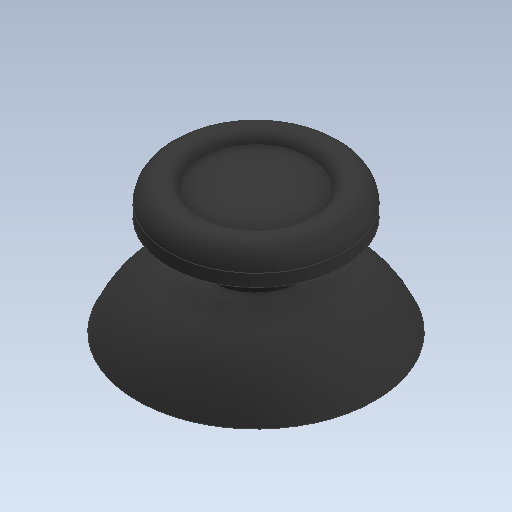
# Autodesk Inventor part: Joystick Cap
Saved by Autodesk Inventor 2020 (Build 240168000, 168)
## iProperties
Created: 2021-03-29
Part Number: Joystick Cap
Material: Generic
Document SubType Name: Modeling
Designer: Luke
Density: 1 g/cm^3
Appearance: Default
Author: Luke
Autodesk Inventor part; units mm, degrees
ref_plane "YZ Plane" through (0, 0, 0) normal (1, 0, 0) x (0, 1, 0)
ref_plane "XZ Plane" through (0, 0, 0) normal (0, 1, 0) x (-1, 0, 0)
ref_plane "XY Plane" through (0, 0, 0) normal (0, 0, 1) x (1, 0, 0)
sketch "Sketch1" plane through (0, 0, 0) normal (0, 1, 0) x (-1, 0, 0)
  line L0 (1.3229, -1.5) -> (-1.3229, -1.5)
  line L1 (-1.3229, 1.5) -> (1.3229, 1.5)
  arc A0 (1.3229, -1.5) -> (1.3229, 1.5) centre (0, 0) ccw
  arc A1 (-1.3229, 1.5) -> (-1.3229, -1.5) centre (0, 0) ccw
  circle A2 centre (0, 0) radius 4.67
  dimension "d1" = 9.34
  constraints: 4 end point, 4 point on circle, 3 centre point, 1 coincident, 1 horizontal, 1 parallel
  measures "d1" diameter of A2
extrude "Extrusion1" add sketch "Sketch1" along normal blind 3.6
sketch "Sketch2" plane through (0, 0, 0) normal (0, 0, 1) x (1, 0, 0)
  line L0 (4.67, 3.6) -> (-4.67, 3.6) projected
  line L1 (0, 3.6) -> (9.08, 3.6)
  line L2 (0, 3.6) -> (9.08, 3.6) construction
  line L3 (0, 3.6) -> (0, 6.9)
  line L4 (9.08, 4.9) -> (9.08, 3.461)
  arc A0 (9.08, 4.9) -> (7.08, 6.9) centre (7.08, 4.9) ccw
  line L5 (0, 6.9) -> (0, 6.17)
  arc A1 (7.08, 6.9) -> (5.535, 6.17) centre (7.08, 4.9) ccw
  arc A2 (5.535, 6.17) -> (0, 6.535) centre (0.5987, -26.5352) ccw
  point P0 (0, 6.535)
  dimension "d5" = 9.08
  dimension "d8" = 3.3
  dimension "d9" = 2
  dimension "d10" = 0.73
  constraints: 10 end point, 7 point on circle, 3 centre point, 2 horizontal, 2 midpoint, 1 concentric, 1 perpendicular, 1 point on line, 1 tangent, 1 vertical
  measures "d5" distance of L1.start L1.end
  measures "d8" distance of L1.start L3.end
  measures "d9" radius of A0
  measures "d10" distance of L3.end L5.end
revolve "Revolution1" add sketch "Sketch2" angle 360 about axis through (0, 3.6, 0) along (0, 1, 0)
sketch "Sketch3" plane through (0, 0, 0) normal (0, 0, 1) x (1, 0, 0)
  arc A0 (12.4, -6.81) -> (4.67, 0) centre (1.8593, -10.9825) ccw
  arc A1 (11.1849, -6.81) -> (4.3923, -1.085) centre (1.8593, -10.9825) ccw
  line L0 (12.4, -6.81) -> (11.1849, -6.81)
  line L1 (2, 0) -> (2, -1.085)
  line L2 (2, -1.085) -> (4.3923, -1.085)
  line L3 (4.67, 0) -> (-4.67, 0) projected
  line L4 (2, 0) -> (4.67, 0)
  line L5 (0, -14.559) -> (0, 10.4765) projected
  point P0 (0, 0)
  dimension "d14" = 1.12
  constraints: 8 end point, 4 point on circle, 2 centre point, 1 collinear, 1 horizontal, 1 perpendicular, 1 vertical
  measures "d14" radial gap between concentric circles of A0 A1
revolve "Revolution2" add sketch "Sketch3" angle 360 about axis through (0, -10, 0) along (0, 1, 0)
sketch "Sketch4" plane through (0, 0, 0) normal (0, -1, 0) x (1, 0, 0)
  arc A0 (-1.3229, -1.5) -> (1.3229, -1.5) centre (0, 0) ccw projected
  line L0 (-1.3229, -1.5) -> (1.3229, -1.5) projected
  arc A1 (1.3229, 1.5) -> (-1.3229, 1.5) centre (0, 0) ccw projected
  line L1 (1.3229, 1.5) -> (-1.3229, 1.5) projected
extrude "Extrusion2" add sketch "Sketch4" along normal up to surface (1.085 mm away)
sketch "Sketch5" plane through (0, -1.085, 0) normal (0, -1, 0) x (1, 0, 0)
  line L0 (-1.3229, -1.5) -> (1.3229, -1.5) projected
  arc A0 (1.3229, -1.5) -> (1.3229, 1.5) centre (0, 0) ccw projected
  line L1 (1.3229, 1.5) -> (-1.3229, 1.5) projected
  arc A1 (-1.3229, 1.5) -> (-1.3229, -1.5) centre (0, 0) ccw projected
extrude "Extrusion3" cut sketch "Sketch5" against normal blind 4.96
body "Solid1"
